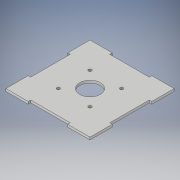
# Autodesk Inventor part: BASE_TECHO
Saved by Autodesk Inventor 2019 (Build 230136000, 136)
## iProperties
Created: 2020-02-12
Part Number: BASE_TECHO
Material: Genérico
Document SubType Name: Modeling
Designer: omar-
Density: 1 g/cm^3
Appearance: Valor por defecto
Author: omar-
Autodesk Inventor part; units mm, degrees
ref_plane "YZ Plane" through (0, 0, 0) normal (1, 0, 0) x (0, 1, 0)
ref_plane "XZ Plane" through (0, 0, 0) normal (0, 1, 0) x (-1, 0, 0)
ref_plane "XY Plane" through (0, 0, 0) normal (0, 0, 1) x (1, 0, 0)
sketch "Boceto1" plane through (0, 0, 0) normal (0, 1, 0) x (-1, 0, 0)
  circle A0 centre (0, 0) radius 13
  line L0 (-53.18, 53.18) -> (53.18, 53.18)
  line L1 (53.18, 53.18) -> (53.18, -53.18)
  line L2 (53.18, -53.18) -> (-53.18, -53.18)
  line L3 (-53.18, -53.18) -> (-53.18, 53.18)
  line L4 (-53.18, 53.18) -> (53.18, -53.18) construction
  line L5 (53.18, 53.18) -> (-53.18, -53.18) construction
  line L6 (25, 53.18) -> (-25, 53.18)
  line L7 (-25, 53.18) -> (-25, 50)
  line L8 (-25, 50) -> (25, 50)
  line L9 (25, 50) -> (25, 53.18)
  line L10 (53.18, 25) -> (50, 25)
  line L11 (50, 25) -> (50, -25)
  line L12 (50, -25) -> (53.18, -25)
  line L13 (53.18, -25) -> (53.18, 25)
  line L14 (25, -50) -> (-25, -50)
  line L15 (-25, -50) -> (-25, -53.18)
  line L16 (-25, -53.18) -> (25, -53.18)
  line L17 (25, -53.18) -> (25, -50)
  line L18 (-50, 25) -> (-53.18, 25)
  line L19 (-53.18, 25) -> (-53.18, -25)
  line L20 (-53.18, -25) -> (-50, -25)
  line L21 (-50, -25) -> (-50, 25)
  circle A1 centre (20, 20) radius 2
  circle A2 centre (20, -20) radius 2
  circle A3 centre (-20, -20) radius 2
  circle A4 centre (-20, 20) radius 2
  dimension "d0" = 26
  dimension "d1" = 106.36
  dimension "d2" = 106.36
  dimension "d3" = 3.18
  dimension "d4" = 50
  dimension "d5" = 25
  dimension "d6" = 25
  dimension "d9" = 4
  dimension "d10" = 4
  dimension "d11" = 4
  dimension "d12" = 4
  dimension "d13" = 20
  dimension "d14" = 20
  dimension "d15" = 40
  dimension "d16" = 20
  dimension "d17" = 40
  dimension "d18" = 40
  dimension "d19" = 40
  constraints: 44 end point, 10 parallel, 6 collinear, 6 equal length, 5 centre point, 5 horizontal, 5 perpendicular, 2 midpoint, 1 coincident, 1 point on line
  measures "d0" diameter of A0
  measures "d1" distance of L1.end L2.end
  measures "d2" distance of L0.end L1.end
  measures "d3" distance of L11.end L12.end
  measures "d4" distance of L10.end L11.end
  measures "d5" distance from line of L9 point (0, 0)
  measures "d6" vertical distance of L10.end A0.centre
  measures "d9" diameter of A1
  measures "d10" diameter of A2
  measures "d11" diameter of A3
  measures "d12" diameter of A4
  measures "d13" horizontal distance of point (0, 0) A1.centre
  measures "d14" horizontal distance of A1.centre point (0, 0)
  measures "d15" distance of A2.centre A1.centre
  measures "d16" horizontal distance of point (0, 0) A2.centre
  measures "d17" distance of A4.centre A1.centre
  measures "d18" distance of A3.centre A4.centre
  measures "d19" distance of A2.centre A3.centre
extrude "Extrusión2" add sketch "Boceto1" along normal blind 3.18 contours L0 L7 L8 L9 L1 L10 L11 L12 L2 L17 L14 L15 L3 L20 L21 L18
